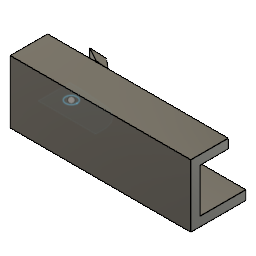
PlayStation Vita Camera Mount v2 (Autodesk Fusion 360 design; units mm, degrees)
Autodesk Fusion 360 part; units mm, degrees
note: some values were not read from the file. Set by a fixed rule: which sketch regions a step uses.
sketch "Sketch1" plane through (0, 0, 0) normal (0, 1, 0) x (1, 0, 0)
  circle A0 centre (0, 0) radius 1.625
  dimension "d8" = 3.25
  constraint coincident A0.centre origin
  measures "d8" diameter of A0
extrude "Extrude1" add sketch "Sketch1" along normal blind 7 makes body 1
sketch "Sketch2" plane through (0, 0, 0) normal (0, -1, 0) x (1, 0, 0)
  circle A0 centre (0, 0) radius 1.625
  line L0 (0, 0) -> (0, -2.125)
  circle A1 centre (0, 1.375) radius 3.5
  dimension "d9" = 2.125
  dimension "d10" = 7
  constraint coincident A0.centre L0.start
  constraint vertical L0
  constraint coincident L0.end A1
  measures "d9" distance of A0.centre L0.end
  measures "d10" diameter of A1
extrude "Extrude2" add sketch "Sketch2" along normal blind 5 contours A0 | A1 bodies 1
sketch "Sketch3" plane through (0, 0, 0) normal (0, 1, 0) x (-1, 0, 0)
  circle A0 centre (0, 1.375) radius 3.5
  circle A1 centre (0, 0) radius 1.625
  line L0 (0, -2.125) -> (12.5, -2.125)
  line L1 (12.5, -2.125) -> (12.5, -3.125)
  line L2 (12.5, -3.125) -> (0, -2.125)
  line L3 (0, -2.125) -> (-8, -2.125)
  line L4 (-8, -2.125) -> (-8, 6.375)
  arc A2 (-8, 6.375) -> (0, -2.125) centre (1.0912, 6.9168) ccw
  line L5 (12.5, -2.125) -> (-8, -2.125)
  line L6 (-8, -2.125) -> (-8, 6.375)
  line L7 (-8, 6.375) -> (12.5, 6.375)
  line L8 (12.5, 6.375) -> (12.5, -2.125)
  dimension "d11" = 12.5
  dimension "d12" = 1
  dimension "d13" = 8
  dimension "d14" = 8.5
  constraint coincident A0 L0.start
  constraint horizontal L0
  constraint perpendicular L0 L1
  constraint horizontal L3
  constraint perpendicular L3 L4
  constraint horizontal L5
  constraint vertical L6
  constraint horizontal L7
  constraint vertical L8
  measures "d11" distance of L0.start L0.end
  measures "d12" distance of L0.end L1.end
  measures "d13" distance of L0.start L3.end
  measures "d14" distance of L3.end L4.end
extrude "Extrude3" add sketch "Sketch3" against normal blind 5 contours A0 L0 A2 L5 L7 L8 | L0 L1 L2 L5 bodies 1
sketch "Sketch4" plane through (0, 7, 0) normal (0, 1, 0) x (-1, 0, 0)
  circle A0 centre (0, 0) radius 1.625
  line L0 (0, 0) -> (-5, 0)
  line L1 (-5, 0) -> (-5, 2)
  line L2 (-5, 2) -> (-1.0307, -1.2563)
  line L3 (-5, 2) -> (0.1201, 1.6206)
  line L4 (0, 0) -> (7, 0)
  line L5 (7, 0) -> (7, -2)
  line L6 (7, -2) -> (-0.0864, -1.6227)
  line L7 (7, -2) -> (0.7839, 1.4234)
  dimension "d17" = 5
  dimension "d18" = 2
  dimension "d19" = 7
  dimension "d20" = 2
  constraint coincident A0.centre L0.start
  constraint horizontal L0
  constraint perpendicular L0 L1
  constraint coincident A0 L2.end
  constraint tangent A0 L2
  constraint coincident A0 L3.end
  constraint tangent A0 L3
  constraint parallel L0 L4
  constraint perpendicular L4 L5
  constraint coincident A0 L6.end
  constraint tangent A0 L6
  constraint coincident A0 L7.end
  constraint tangent A0 L7
  measures "d17" distance of A0.centre L0.end
  measures "d18" distance of L0.end L1.end
  measures "d19" distance of A0.centre L4.end
  measures "d20" distance of L4.end L5.end
extrude "Extrude4" add sketch "Sketch4" against normal blind 7 contours A0 L4 L6 L7 | A0 L4 L7 | A0 L0 L2 L3 | A0 L0 L2 bodies 1
extrude "Extrude5" add 1 faces at (-1.5, -5, 3.5417) along direction (0, -1, 0) blind 6.25 on bodies 1 bodies 1
extrude "Extrude6" add 1 faces at (1.1667, -3.75, 6.375) along direction (0, 0, 1) blind 4 on bodies 1 bodies 1
extrude "Extrude7" add 1 faces at (-12.5, -7.5, 1.375) along direction (-1, 0, 0) blind 4 on bodies 1 bodies 1
sketch "Sketch5" plane through (0, 0, 10.375) normal (0, 0, 1) x (1, 0, 0)
  line L0 (8, 0) -> (-16.5, 0)
  line L1 (-16.5, 0) -> (-16.5, -11.25)
  line L2 (-16.5, -11.25) -> (8, -11.25)
  line L3 (8, -11.25) -> (8, 0)
  line L4 (-16.5, -5.625) -> (-14.5, -5.625)
  line L5 (-14.5, -5.625) -> (-14.5, -4.025)
  line L6 (-14.5, -4.025) -> (-5, -4.025)
  line L7 (-5, -4.025) -> (-5, -7.225)
  line L8 (-5, -7.225) -> (-14.5, -7.225)
  line L9 (-14.5, -7.225) -> (-14.5, -4.025)
  dimension "d29" = 2
  dimension "d30" = 1.6
  dimension "d31" = 3.2
  dimension "d32" = 9.5
  constraint midpoint L1 L4.start
  constraint perpendicular L1 L4
  constraint perpendicular L4 L5
  constraint horizontal L6
  constraint vertical L7
  constraint horizontal L8
  constraint vertical L9
  measures "d29" distance of L4.start L4.end
  measures "d30" distance of L4.end L5.end
  measures "d31" distance of L5.end L8.end
  measures "d32" distance of L5.end L6.end
extrude "Extrude8" cut sketch "Sketch5" against normal blind 12.7 contours L5 L6 L7 L8 L9 bodies 1
sketch "Sketch6" plane through (0, -7.225, 0) normal (0, 1, 0) x (-1, 0, 0)
  line L0 (14.5, 10.375) -> (5, 10.375)
  line L1 (5, 10.375) -> (5, -2.325)
  line L2 (5, -2.325) -> (14.5, -2.325)
  line L3 (14.5, -2.325) -> (14.5, 10.375)
  line L4 (9.75, -2.325) -> (9.75, 8.375)
  circle A0 centre (9.75, 3.025) radius 2.4
  dimension "d35" = 10.7
  dimension "d36" = 4.8
  constraint midpoint L2 L4.start
  constraint perpendicular L2 L4
  constraint midpoint L4 A0.centre
  measures "d35" distance of L4.start L4.end
  measures "d36" diameter of A0
extrude "Extrude9" cut sketch "Sketch6" against normal blind 6 contours L4 A0 | L4 A0 bodies 1
sketch "Sketch7" plane through (0, -11.25, 0) normal (0, -1, 0) x (1, 0, 0)
  circle A0 centre (-9.75, 3.025) radius 2.4
  arc A1 (0, -2.125) -> (1.3269, -1.8637) centre (0, 1.375) ccw
  arc A2 (1.3269, -1.8637) -> (8, 6.375) centre (-1.0912, 6.9168) ccw
  line L0 (8, 6.375) -> (8, 10.375)
  line L1 (8, 10.375) -> (-16.5, 10.375)
  line L2 (-16.5, 10.375) -> (-16.5, -3.125)
  line L3 (-16.5, -3.125) -> (-12.5, -3.125)
  line L4 (-12.5, -3.125) -> (0, -2.125)
  circle A3 centre (-9.75, 3.025) radius 2.4
  constraint concentric A0 A3
extrude "Extrude10" cut sketch "Sketch7" against normal blind 9.25 contours A0 A3 bodies 1
sketch "Sketch8" plane through (-16.5, 0, 0) normal (-1, 0, 0) x (0, 0, 1)
  line L0 (10.375, 0) -> (-3.125, 0)
  line L1 (-3.125, 0) -> (-3.125, -11.25)
  line L2 (-3.125, -11.25) -> (10.375, -11.25)
  line L3 (10.375, -11.25) -> (10.375, 0)
  line L4 (10.375, -11.25) -> (12.375, -11.25)
  line L5 (12.375, -11.25) -> (12.375, -13.25)
  line L6 (12.375, -13.25) -> (10.375, -13.25)
  line L7 (10.375, -13.25) -> (10.375, -11.25)
  line L8 (12.375, -13.25) -> (16.375, -13.25)
  line L9 (16.375, -13.25) -> (16.375, 5.5)
  line L10 (16.375, 5.5) -> (12.375, 5.5)
  line L11 (12.375, 5.5) -> (12.375, -13.25)
  line L12 (16.375, -13.25) -> (-3.125, -13.25)
  line L13 (-3.125, -13.25) -> (-3.125, -17.25)
  line L14 (-3.125, -17.25) -> (16.375, -17.25)
  line L15 (16.375, -17.25) -> (16.375, -13.25)
  line L16 (16.375, 5.5) -> (4.375, 5.5)
  line L17 (4.375, 5.5) -> (4.375, 9.5)
  line L18 (4.375, 9.5) -> (16.375, 9.5)
  line L19 (16.375, 9.5) -> (16.375, 5.5)
  dimension "d41" = 2
  dimension "d42" = 2
  dimension "d43" = 18.75
  dimension "d44" = 4
  dimension "d45" = 4
  dimension "d46" = 4
  dimension "d47" = 12
  constraint horizontal L4
  constraint vertical L5
  constraint horizontal L6
  constraint vertical L7
  constraint coincident L2.end L3.start
  constraint horizontal L8
  constraint vertical L9
  constraint horizontal L10
  constraint vertical L11
  constraint horizontal L12
  constraint vertical L13
  constraint horizontal L14
  constraint vertical L15
  constraint horizontal L16
  constraint vertical L17
  constraint horizontal L18
  constraint vertical L19
  measures "d41" distance of L2.end L4.end
  measures "d42" distance of L2.end L6.end
  measures "d43" distance of L5.end L10.end
  measures "d44" distance of L5.end L8.end
  measures "d45" distance of L8.end L14.end
  measures "d46" distance of L9.end L18.end
  measures "d47" distance of L9.end L16.end
extrude "Extrude11" add sketch "Sketch8" along normal blind 10 separate body contours L5 L8 L9 L10 L11 L12 L16 | L6 L8 L12 L13 L14 L15 | L10 L16 L17 L18 L19 makes body 2
extrude "Extrude12" add 1 faces at (-16.5, -15.9167, 7.875) along direction (1, 0, 0) blind 75 on bodies 2 bodies 2
extrude "Extrude13" cut 1 faces at (-26.5, -7, 15.0417) along direction (1, 0, 0) blind 10 on bodies 2 bodies 2
extrude "Extrude14" cut sketch "Sketch7" along normal blind 6 contours A0 A3 bodies 2
move_face "MoveFace1" to x (1, 0, 0) y (0, 1, 0) z (0, 0, 1) at (-0.2029, 0, 1.9897) 1 faces at (-7.3619, -14.5833, 3.264) on bodies 2
extrude "Extrude15" add 1 faces at (-16.5, -7, 15.0417) along direction (-1, 0, 0) blind 2 on bodies 2 bodies 2
sketch "Sketch9" plane through (0, -17.25, 0) normal (0, -1, 0) x (1, 0, 0)
  circle A0 centre (-9.9529, 5.0147) radius 2.4
  line L0 (-18.5, -3.125) -> (58.5, -3.125)
  line L1 (58.5, -3.125) -> (58.5, 16.375)
  line L2 (58.5, 16.375) -> (-18.5, 16.375)
  line L3 (-18.5, 16.375) -> (-18.5, -3.125)
  circle A1 centre (-9.9529, 5.0147) radius 4.375
  dimension "d58" = 8.75
  constraint concentric A0 A1
  measures "d58" diameter of A1
extrude "Extrude16" add sketch "Sketch9" along normal blind 1.5 contours A1 bodies 2
extrude "Extrude17" cut 1 faces at (-6.2525, -18.75, 4.7973) along direction (0, 1, 0) blind 3 on bodies 2 bodies 2
chamfer "Chamfer1" distance 1.95 angle 45 1 edges at (-12.1905, -15.75, 4.1468) on bodies 2
move_face "MoveFace2" by (0, 0, 4) 2 faces at (7.1667, -0.75, 12.375) (7.1667, 0.5833, 16.375) on bodies 2
equation "d9 = 1.625 mm + 0.5 mm"
equation "d39 = -11.25 mm + 2 mm"
